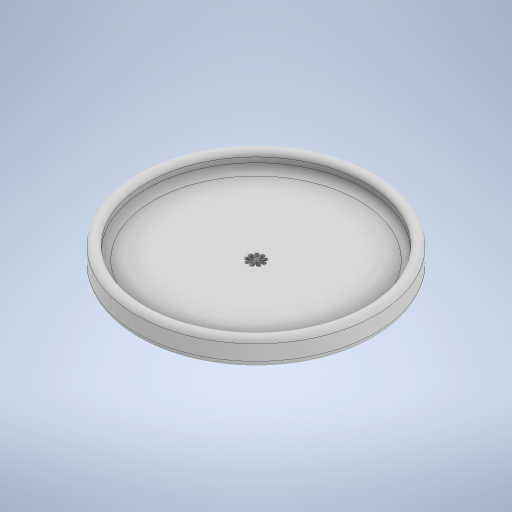
# Autodesk Inventor part: Orchid Coaster V4
Saved by Autodesk Inventor 2024 (Build 280153000, 153)
## iProperties
Created: 2024-02-28
Part Number: Orchid Coaster V4
Material: Generic
Document SubType Name: Modeling
Designer: haque
Density: 1 g/cm^3
Appearance: Default
Author: haque
Autodesk Inventor part; units mm, degrees
ref_plane "YZ Plane" through (0, 0, 0) normal (1, 0, 0) x (0, 1, 0)
ref_plane "XZ Plane" through (0, 0, 0) normal (0, 1, 0) x (-1, 0, 0)
ref_plane "XY Plane" through (0, 0, 0) normal (0, 0, 1) x (1, 0, 0)
sketch "Sketch1" plane through (0, 0, 0) normal (0, 1, 0) x (-1, 0, 0)
  circle A0 centre (0, 0) radius 32.5
  circle A1 centre (0, 0) radius 35.5
  dimension "d0" = 65
  dimension "d1" = 71
  constraints: 2 centre point, 2 coincident
  measures "d0" diameter of A0
  measures "d1" diameter of A1
extrude "Extrusion1" add sketch "Sketch1" along normal blind 8
extrude "Extrusion2" add sketch "Sketch1" along normal blind 3 contours A0
fillet "Fillet1" radius 2 2 edges at (35.5, 0, 0) (32.5, 3, 0)
fillet "Fillet2" radius 1.5 2 edges at (32.5, 8, 0) (35.5, 8, 0)
sketch "Sketch2" plane through (0, 3, 0) normal (0, 1, 0) x (1, 0, 0)
  circle A0 centre (0, 0) radius 0.25
  circle A1 centre (0, 0) radius 2.5
  circle A2 centre (0, 2) radius 0.5
  line L0 (-0.5, 2) -> (-0.5, 1.5) construction
  line L1 (-0.5, 1.5) -> (-0.25, 0.892563) construction
  line L2 (-0.25, 0.892563) -> (0, 0.421283) construction
  spline S0 degree 3 poles (-0.5, 2) (-0.5, 1.5) (-0.25, 0.892563) (0, 0.421283) knots 1 1 1 1 2 2 2 2
  line L3 (-0.5, 1.5) -> (0.5, 1.5)
  line L4 (-0.25, 0.892563) -> (0.25, 0.892563)
  line L5 (0.5, 2) -> (0.5, 1.5) construction
  line L6 (0.5, 1.5) -> (0.25, 0.892563) construction
  line L7 (0.25, 0.892563) -> (0, 0.421283) construction
  spline S1 degree 3 poles (0.5, 2) (0.5, 1.5) (0.25, 0.892563) (0, 0.421283) knots 1 1 1 1 2 2 2 2
  dimension "d12" = 0.5
  dimension "d13" = 5
  constraints: 6 coincident, 4 end point, 3 centre point, 2 horizontal, 2 point on circle, 2 tangent, 2 vertical, 6 other
  measures "d12" diameter of A0
  measures "d13" diameter of A1
sketch "Sketch2 outline for Extrusion4" plane through (0, 3, 0) normal (0, 1, 0) x (1, 0, 0)
  circle A0 centre (0, 0) radius 0.25
  spline S0 degree 3 poles (0.5, 2) (0.5, 1.5) (0.25, 0.892563) (0, 0.421283) knots 0 0 0 0 1 1 1 1
  spline S1 degree 3 poles (-0.5, 2) (-0.5, 1.5) (-0.25, 0.892563) (0, 0.421283) knots 0 0 0 0 1 1 1 1
  arc A1 (0.5, 2) -> (-0.5, 2) centre (0, 2) ccw
extrude "Extrusion4" cut sketch "Sketch2 outline for Extrusion4" against normal blind 1
pattern_circular "Circular Pattern1" count 9 over 360 about axis through (0, -10, 0) along (0, 1, 0) of "Extrusion4"
body "Solid1"
